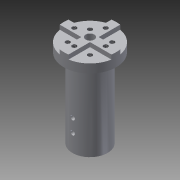
# Autodesk Inventor part: Achse
Saved by Autodesk Inventor 2013 (Build 170138000, 138)
## iProperties
Created: 2012-12-21
Part Number: Achse
Material: Aluminium 6061
Document SubType Name: Modeling
Designer: Lukas
Density: 1 g/cm^3
Author: Lukas
Autodesk Inventor part; units mm, degrees
ref_plane "YZ Plane" through (0, 0, 0) normal (1, 0, 0) x (0, 1, 0)
ref_plane "XZ Plane" through (0, 0, 0) normal (0, 1, 0) x (-1, 0, 0)
ref_plane "XY Plane" through (0, 0, 0) normal (0, 0, 1) x (1, 0, 0)
sketch "Skizze1" plane through (0, 0, 0) normal (1, 0, 0) x (0, 1, 0)
  line L0 (0, 0) -> (20, 0)
  line L1 (20, 0) -> (20, 10)
  line L2 (20, 10) -> (0, 10)
  line L3 (0, 10) -> (0, 0)
  line L4 (0, 10) -> (20, 10)
  line L5 (20, 10) -> (20, 90)
  line L6 (20, 90) -> (0, 90)
  line L7 (0, 90) -> (0, 10)
  line L8 (0, 90) -> (30, 90)
  line L9 (30, 90) -> (30, 100)
  line L10 (30, 100) -> (0, 100)
  line L11 (0, 100) -> (0, 90)
  dimension "d0" = 20
  dimension "d1" = 10
  dimension "d2" = 20
  dimension "d3" = 80
  dimension "d4" = 30
  dimension "d5" = 10
  constraints: 24 end point, 6 parallel, 3 horizontal, 3 perpendicular
  measures "d0" distance of L2.end L1.end
  measures "d1" distance of L1.end L0.end
  measures "d2" distance of L6.end L5.end
  measures "d3" distance of L5.end L4.end
  measures "d4" distance of L10.end L9.end
  measures "d5" distance of L9.end L8.end
revolve "Umdrehung1" add sketch "Skizze1" angle 360 about axis through (0, 0, 90) along (0, 0, -1)
sketch "Skizze5" plane through (0, 0, 100) normal (0, 0, 1) x (1, 0, 0)
  circle A0 centre (0, 0) radius 30 projected
  line L0 (5, 5) -> (29.5804, 5)
  line L1 (5, -5) -> (29.5804, -5)
  line L2 (5, -5) -> (5, -29.5804)
  line L3 (5, 5) -> (5, 29.5804)
  line L4 (-5, 5) -> (-5, 29.5804)
  line L5 (-5, 5) -> (-29.5804, 5)
  line L6 (-5, -5) -> (-29.5804, -5)
  line L7 (-5, -5) -> (-5, -29.5804)
  arc A1 (5, 29.5804) -> (-5, 29.5804) centre (0, 0) ccw
  arc A2 (29.5804, -5) -> (29.5804, 5) centre (0, 0) ccw
  arc A3 (-5, -29.5804) -> (5, -29.5804) centre (0, 0) ccw
  arc A4 (-29.5804, 5) -> (-29.5804, -5) centre (0, 0) ccw
  constraints: 16 end point, 8 point on circle, 4 centre point, 4 coincident, 3 equal length, 3 perpendicular, 1 horizontal, 10 other
extrude "Extrusion3" add sketch "Skizze5" along normal blind 5 contours A0 L1 L2 L7 L6 L5 L4 L3 L0
sketch "Skizze6" plane through (0, 0, 105) normal (0, 0, 1) x (1, 0, 0)
  arc A0 (29.5804, -5) -> (29.5804, 5) centre (0, 0) ccw projected
  circle A1 centre (0, 0) radius 5
  dimension "d19" = 10
  constraints: 1 centre point, 1 coincident
  measures "d19" diameter of A1
extrude "Extrusion4" cut sketch "Skizze6" against normal blind 95
sketch "Skizze7" plane through (0, 0, 105) normal (0, 0, 1) x (1, 0, 0)
  circle A0 centre (0, 0) radius 5 projected
  point P0 (0, 18)
  point P1 (18, 0)
  point P2 (0, -18)
  point P3 (-18, 0)
  dimension "d22" = 18
  dimension "d23" = 18
  dimension "d24" = 18
  dimension "d25" = 18
  measures "d22" distance of point (0, 18) A0.centre
  measures "d23" distance of point (18, 0) A0.centre
  measures "d24" distance of point (0, -18) A0.centre
  measures "d25" distance of point (-18, 0) A0.centre
hole "Bohrung1" at (0, 18, 105) at (18, 0, 105) at (0, -18, 105) at (-18, 0, 105) direction (0, 0, -1) diameter 5 depth 12 tip angle 118
sketch "Skizze8" plane through (5, -5, 100) normal (0, 0, 1) x (1, 0, 0)
  arc A0 (0, -24.5804) -> (24.5804, 0) centre (-5, 5) ccw projected
  circle A1 centre (-5, 5) radius 18
  line L0 (-5, 5) -> (7.7279, 17.7279)
  line L1 (-5, 5) -> (13, 5) construction
  line L2 (-5, 5) -> (7.7279, -7.7279)
  line L3 (-5, 5) -> (-17.7279, -7.7279)
  line L4 (-5, 5) -> (-17.7279, 17.7279)
  dimension "d33" = 36
  dimension "d34" = 45
  constraints: 10 end point, 5 coincident, 4 point on circle, 3 perpendicular, 1 centre point, 1 equal length, 1 horizontal
  measures "d33" diameter of A1
  measures "d34" angle of L1 L0
hole "Bohrung2" at (-12.7279, -12.7279, 100) at (12.7279, -12.7279, 100) at (12.7279, 12.7279, 100) at (-12.7279, 12.7279, 100) direction (0, 0, -1) diameter 5 depth 8 tip angle 118
thread "Gewinde1" size "M5x0.8" class "6H" standard "ANSI Metric M Profile" full length
thread "Gewinde2" size "M5x0.8" class "6H" standard "ANSI Metric M Profile" full length
thread "Gewinde3" size "M5x0.8" class "6H" standard "ANSI Metric M Profile" full length
thread "Gewinde4" size "M5x0.8" class "6H" standard "ANSI Metric M Profile" full length
thread "Gewinde5" size "M5x0.8" class "6H" standard "ANSI Metric M Profile" full length
thread "Gewinde6" size "M5x0.8" class "6H" standard "ANSI Metric M Profile" full length
thread "Gewinde7" size "M5x0.8" class "6H" standard "ANSI Metric M Profile" full length
thread "Gewinde8" size "M5x0.8" class "6H" standard "ANSI Metric M Profile" full length
sketch "Skizze9" plane through (0, 0, 105) normal (0, 0, 1) x (1, 0, 0)
  point P0 (0, 18)
  point P1 (-18, 0)
  point P2 (0, -18)
  point P3 (18, 0)
hole "Bohrung3" at (0, 18, 105) at (-18, 0, 105) at (0, -18, 105) at (18, 0, 105) direction (0, 0, -1) diameter 4.134 depth 14.3144 tip angle 120 thread size "M5x0.8" class "6H" standard "ISO Metric profile"
sketch "Skizze10" plane through (5, -5, 100) normal (0, 0, 1) x (1, 0, 0)
  point P0 (7.7279, 17.7279)
  point P1 (-17.7279, 17.7279)
  point P2 (-17.7279, -7.7279)
  point P3 (7.7279, -7.7279)
  point P4 (-17.7279, -7.7279)
hole "Bohrung5" at (12.7279, 12.7279, 100) at (-12.7279, 12.7279, 100) at (-12.7279, -12.7279, 100) at (12.7279, -12.7279, 100) at (-12.7279, -12.7279, 100) direction (0, 0, -1) diameter 4.134 depth 9.3144 tip angle 120 thread size "M5x0.8" class "6H" standard "ISO Metric profile"
ref_plane "Arbeitsebene1" through (0, 20, 5) normal (0, -1, 0) x (1, 0, 0)
sketch "Skizze13" plane through (0, 20, 5) normal (0, -1, 0) x (1, 0, 0)
  line L0 (-20, -5) -> (20, -5) projected
  point P0 (0, -5)
  point P1 (0, 15)
  point P2 (0, 30)
  dimension "d93" = 20
  dimension "d94" = 15
  measures "d93" distance from line of L0 point (0, 15)
  measures "d94" distance of point (0, 30) point (0, 15)
hole "Bohrung12" at (0, 20, 20) at (0, 20, 35) direction (0, -1, 0) diameter 5 end through all
sketch "Skizze11" plane through (5, -5, 100) normal (0, 0, 1) x (1, 0, 0)
  point P0 (7.7279, 17.7279)
  point P1 (-17.7279, 17.7279)
  point P2 (-17.7279, -7.7279)
  point P3 (7.7279, -7.7279)
  point P4 (-17.7279, -7.7279)
sketch "Skizze12" plane through (0, 0, 105) normal (0, 0, 1) x (1, 0, 0)
  point P0 (0, 18)
  point P1 (-18, 0)
  point P2 (0, -18)
  point P3 (18, 0)
sketch "Skizze14" plane through (5, 5, 100) normal (0, 0, 1) x (1, 0, 0)
  point P0 (-5, 13)
  point P1 (-23, -5)
  point P2 (-5, -23)
  point P3 (13, -5)
sketch "Skizze15" plane through (-29.5804, 5, 100) normal (0, 0, 1) x (1, 0, 0)
  point P0 (42.3083, 7.7279)
  point P1 (16.8525, 7.7279)
  point P2 (16.8525, -17.7279)
  point P3 (42.3083, -17.7279)
  point P4 (16.8525, -17.7279)
